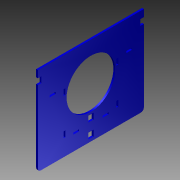
# Autodesk Inventor part: OpenROV 2_3 Dev Top
Saved by Autodesk Inventor 2012 (Build 160160000, 160)
## iProperties
Created: 2011-09-22
Part Number: OpenROV 2_3 Dev Top
Document SubType Name: Modeling
Designer: user
Density: 1 g/cm^3
Material: Default
Author: user
Autodesk Inventor part; units mm, degrees
ref_plane "YZ Plane" through (0, 0, 0) normal (1, 0, 0) x (0, 1, 0)
ref_plane "XZ Plane" through (0, 0, 0) normal (0, 1, 0) x (-1, 0, 0)
ref_plane "XY Plane" through (0, 0, 0) normal (0, 0, 1) x (1, 0, 0)
sketch "Sketch2" plane through (0, 0, 0) normal (0, 1, 0) x (-1, 0, 0)
  line L0 (90, -53) -> (84, -53)
  line L1 (84, -53) -> (84, -43)
  line L2 (84, -43) -> (90, -43)
  line L3 (-90, -53) -> (-84, -53)
  line L4 (-84, -53) -> (-84, -43)
  line L5 (-84, -43) -> (-90, -43)
  line L6 (70, -18) -> (60, -18)
  line L7 (60, -18) -> (60, -15)
  line L8 (60, -15) -> (70, -15)
  line L9 (70, -15) -> (70, -18)
  line L10 (-70, -18) -> (-60, -18)
  line L11 (-60, -18) -> (-60, -15)
  line L12 (-60, -15) -> (-70, -15)
  line L13 (-70, -15) -> (-70, -18)
  circle A0 centre (0, 0) radius 41.275
  line L14 (46.5, -15) -> (43.5, -15)
  line L15 (43.5, -15) -> (43.5, -5)
  line L16 (43.5, -5) -> (46.5, -5)
  line L17 (46.5, -5) -> (46.5, -15)
  line L18 (-46.5, -15) -> (-43.5, -15)
  line L19 (-43.5, -15) -> (-43.5, -5)
  line L20 (-43.5, -5) -> (-46.5, -5)
  line L21 (-46.5, -5) -> (-46.5, -15)
  line L22 (43.5, 57) -> (43.5, 47)
  line L23 (43.5, 47) -> (46.5, 47)
  line L24 (46.5, 47) -> (46.5, 57)
  line L25 (-46.5, 47) -> (-43.5, 47)
  line L26 (-43.5, 47) -> (-43.5, 57)
  line L27 (-46.5, 57) -> (-46.5, 47)
  line L28 (-85, 85) -> (85, 85)
  arc A1 (-85, 85) -> (-90, 80) centre (-85, 80) ccw
  arc A2 (90, 80) -> (85, 85) centre (85, 80) ccw
  line L29 (46.5, 57) -> (43.5, 57)
  line L30 (-43.5, 57) -> (-46.5, 57)
  line L31 (30, 57) -> (20, 57)
  line L32 (20, 57) -> (20, 60)
  line L33 (20, 60) -> (30, 60)
  line L34 (30, 60) -> (30, 57)
  line L35 (-20, 57) -> (-30, 57)
  line L36 (-30, 57) -> (-30, 60)
  line L37 (-30, 60) -> (-20, 60)
  line L38 (-20, 60) -> (-20, 57)
  line L39 (4.5, 70) -> (-4.5, 70)
  line L40 (-4.5, 70) -> (-4.5, 80)
  line L41 (-4.5, 80) -> (4.5, 80)
  line L42 (4.5, 80) -> (4.5, 70)
  line L43 (4.5, 45) -> (-4.5, 45)
  line L44 (-4.5, 45) -> (-4.5, 55)
  line L45 (-4.5, 55) -> (4.5, 55)
  line L46 (4.5, 55) -> (4.5, 45)
  line L47 (-90, -43) -> (-90, 80)
  line L48 (90, 80) -> (90, -43)
  line L49 (90, -53) -> (90, -65)
  line L50 (-90, -53) -> (-90, -65)
  line L51 (90, -65) -> (-90, -65)
  point P0 (90, 85)
  dimension "d21" = 6
  dimension "d22" = 10
  dimension "d25" = 6
  dimension "d26" = 10
  dimension "d31" = 3
  dimension "d32" = 10
  dimension "d35" = 3
  dimension "d36" = 10
  dimension "d39" = 25
  dimension "d40" = 25
  dimension "d43" = 82.55
  dimension "d52" = 3
  dimension "d53" = 10
  dimension "d54" = 10
  dimension "d55" = 3
  dimension "d58" = 10
  dimension "d59" = 3
  dimension "d62" = 3
  dimension "d65" = 180
  dimension "d66" = 150
  dimension "d90" = 90
  dimension "d91" = 90
  dimension "d103" = 10
  dimension "d104" = 10
  dimension "d108" = 3
  dimension "d109" = 10
  dimension "d110" = 20
  dimension "d111" = 3
  dimension "d112" = 10
  dimension "d113" = 20
  dimension "d114" = 5
  dimension "d115" = 10
  dimension "d116" = 9
  dimension "d117" = 4.5
  dimension "d118" = 10
  dimension "d119" = 9
  dimension "d120" = 15
  dimension "d121" = 4.5
  dimension "d127" = 180
  dimension "d128" = 150
  dimension "d130" = 85.5
  dimension "d131" = 43.5
  dimension "d132" = 43.5
  dimension "d133" = 60
  dimension "d134" = 60
  dimension "d135" = 43.5
  dimension "d136" = 43.5
  dimension "d137" = 90
  dimension "d138" = 28
  dimension "d140" = 47
  dimension "d141" = 47
  constraints: 104 end point, 22 parallel, 12 perpendicular, 11 horizontal, 4 point on circle, 4 tangent, 3 centre point, 2 collinear, 1 point on line
  measures "d21" distance of L0.start L0.end
  measures "d22" distance of L2.end L0.start
  measures "d25" distance of L4.end L5.end
  measures "d26" distance of L5.end L3.start
  measures "d31" distance between parallel lines of L6 L8
  measures "d32" distance between parallel lines of L7 L9
  measures "d35" distance between parallel lines of L12 L10
  measures "d36" distance between parallel lines of L13 L11
  measures "d39" distance between parallel lines of L6 L2
  measures "d40" distance between parallel lines of L10 L5
  measures "d43" diameter of A0
  measures "d52" distance between parallel lines of L15 L17
  measures "d53" distance between parallel lines of L16 L14
  measures "d54" distance of L20.end L18.start
  measures "d55" distance of L19.end L20.end
  measures "d58" distance of L23.end L24.end
  measures "d59" distance of L22.end L23.end
  measures "d62" distance of L25.start L25.end
  measures "d65" distance of L49.end L50.end
  measures "d66" distance of point (90, 85) L49.end
  measures "d90" distance between parallel lines of L28 L16
  measures "d91" distance between parallel lines of L28 L20
  measures "d103" distance between parallel lines of L16 L8
  measures "d104" distance between parallel lines of L20 L12
  measures "d108" distance of L33.end L31.start
  measures "d109" distance of L31.start L31.end
  measures "d110" distance from line of A0.centre L32
  measures "d111" distance of L37.end L35.start
  measures "d112" distance of L35.start L35.end
  measures "d113" distance from line of A0.centre L38
  measures "d114" distance between parallel lines of L28 L41
  measures "d115" distance of L39.end L40.end
  measures "d116" distance of L40.end L41.end
  measures "d117" distance from line of A0.centre L42
  measures "d118" distance of L45.end L43.start
  measures "d119" distance of L43.start L43.end
  measures "d120" distance between parallel lines of L39 L45
  measures "d121" distance from line of L46 A0.centre
  measures "d127" distance between parallel lines of L48 L47
  measures "d128" distance between parallel lines of L51 L28
  measures "d130" distance between parallel lines of L40 L47
  measures "d131" distance from line of A0.centre L15
  measures "d132" distance from line of A0.centre L19
  measures "d133" horizontal distance of A0.centre L11.end
  measures "d134" horizontal distance of A0.centre L7.end
  measures "d135" distance from line of A0.centre L22
  measures "d136" distance from line of A0.centre L26
  measures "d137" angle of L23 L22
  measures "d138" distance between parallel lines of L28 L30
  measures "d140" distance from line of A0.centre L25
  measures "d141" distance from line of A0.centre L23
extrude "Extrusion6" add sketch "Sketch2" along normal blind 3
body "Solid6"
